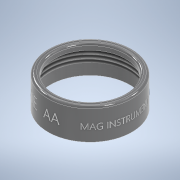
# Autodesk Inventor part: Cap
Saved by Autodesk Inventor 2021 (Build 250183000, 183)
## iProperties
Created: 2020-04-08
Part Number: Cap
Material: Generic
Document SubType Name: Modeling
Designer: Elijah
Density: 1 g/cm^3
Appearance: Silicon Nitride - Polished
Author: Elijah
Autodesk Inventor part; units mm, degrees
ref_plane "XZ Plane" through (0, 0, 0) normal (0, 1, 0) x (-1, 0, 0)
ref_plane "XY Plane" through (0, 0, 0) normal (0, 0, 1) x (1, 0, 0)
sketch "Sketch1" plane through (0, 0, 0) normal (0, 1, 0) x (-1, 0, 0)
  circle A0 centre (0, 0) radius 11.43
  circle A1 centre (0, 0) radius 13.5
  dimension "d0" = 22.86
  dimension "d1" = 27
  constraints: 2 centre point, 2 coincident
  measures "d0" diameter of A0
  measures "d1" diameter of A1
extrude "Extrusion1" add sketch "Sketch1" along normal blind 10
fillet "Fillet1" radius 0.7 2 edges at (13.5, 10, 0) (11.43, 10, 0)
sketch "Sketch2" plane through (0, 0, 0) normal (0, -1, 0) x (1, 0, 0)
  circle A0 centre (0, 0) radius 12.8492
  constraints: 1 centre point, 1 coincident
extrude "Extrusion2" cut sketch "Sketch2" against normal blind 8
ref_plane "Work Plane1" through (13.5, 0, 0) normal (1, 0, 0) x (0, 1, 0)
sketch "Sketch3" plane through (13.5, 0, 0) normal (1, 0, 0) x (0, 1, 0)
  line L0 (7.7302, 43.5284) -> (7.7302, 29.5201) construction
  line L1 (7.7302, 29.5201) -> (-6.2781, 29.5201) construction
  line L2 (-6.2781, 29.5201) -> (-6.2781, 43.5284) construction
  line L3 (-6.2781, 43.5284) -> (7.7302, 43.5284) construction
  line L4 (29.5152, 13.7326) -> (63.5734, 13.7326)
  line L5 (3.4122, 40.2417) -> (5.7555, 40.2417)
  spline S0 degree 2 poles (5.7555, 40.2417) (5.8412, 40.2417) (6.2425, 40.2172) knots 0 0 0 1 1 1
  line L6 (6.2425, 40.2172) -> (6.2425, 40.2264)
  spline S1 degree 2 poles (6.2425, 40.2264) (6.0556, 40.2968) (5.9546, 40.3459) knots 0 0 0 1 1 1
  line L7 (5.9546, 40.3459) -> (3.4122, 41.5221)
  line L8 (3.4122, 41.5221) -> (3.4122, 41.5956)
  line L9 (3.4122, 41.5956) -> (5.9392, 42.7749)
  spline S2 degree 2 poles (5.9392, 42.7749) (6.0618, 42.8331) (6.2517, 42.8821) knots 0 0 0 1 1 1
  line L10 (6.2517, 42.8821) -> (6.2517, 42.8943)
  spline S3 degree 2 poles (6.2517, 42.8943) (6.0311, 42.879) (5.8106, 42.879) knots 0 0 0 1 1 1
  line L11 (5.8106, 42.879) -> (3.4122, 42.879)
  line L12 (3.4122, 42.879) -> (3.4122, 43.1057)
  line L13 (3.4122, 43.1057) -> (6.7142, 43.1057)
  line L14 (6.7142, 43.1057) -> (6.7142, 42.8943)
  line L15 (6.7142, 42.8943) -> (4.0555, 41.663)
  spline S4 degree 2 poles (4.0555, 41.663) (4.0309, 41.6507) (3.9911, 41.6354) knots 0 0 0 1 1 1
  spline S5 degree 2 poles (3.9911, 41.6354) (3.9544, 41.6232) (3.9145, 41.6078) knots 0 0 0 1 1 1
  spline S6 degree 2 poles (3.9145, 41.6078) (3.8533, 41.5833) (3.7798, 41.5588) knots 0 0 0 1 1 1
  line L16 (3.7798, 41.5588) -> (3.7798, 41.5435)
  line L17 (3.7798, 41.5435) -> (3.8533, 41.519)
  spline S7 degree 2 poles (3.8533, 41.519) (3.8625, 41.516) (4.0738, 41.4394) knots 0 0 0 1 1 1
  line L18 (4.0738, 41.4394) -> (6.7142, 40.2264)
  line L19 (6.7142, 40.2264) -> (6.7142, 40.0242)
  line L20 (6.7142, 40.0242) -> (3.4122, 40.0242)
  line L21 (3.4122, 40.0242) -> (3.4122, 40.2417)
  line L22 (3.4122, 37.0194) -> (4.4414, 37.3992)
  line L23 (4.4414, 37.3992) -> (4.4414, 38.8327)
  line L24 (4.4414, 38.8327) -> (3.4122, 39.2125)
  line L25 (3.4122, 39.2125) -> (3.4122, 39.4637)
  line L26 (3.4122, 39.4637) -> (6.7142, 38.217)
  line L27 (6.7142, 38.217) -> (6.7142, 37.9995)
  line L28 (6.7142, 37.9995) -> (3.4122, 36.7651)
  line L29 (3.4122, 36.7651) -> (3.4122, 37.0194)
  spline S8 degree 2 poles (6.1751, 38.0363) (6.2456, 38.0608) (6.3129, 38.0761) knots 0 0 0 1 1 1
  spline S9 degree 2 poles (6.3129, 38.0761) (6.3681, 38.0945) (6.4263, 38.1129) knots 0 0 0 1 1 1
  line L30 (6.4263, 38.1129) -> (6.4263, 38.1221)
  spline S10 degree 2 poles (6.4263, 38.1221) (6.2731, 38.1619) (6.1812, 38.1986) knots 0 0 0 1 1 1
  line L31 (6.1812, 38.1986) -> (4.6497, 38.7531)
  line L32 (4.6497, 38.7531) -> (4.6497, 37.4788)
  line L33 (4.6497, 37.4788) -> (6.1751, 38.0363)
  spline S11 degree 2 poles (3.6419, 33.8184) (3.354, 34.33) (3.354, 34.8721) knots 0 0 0 1 1 1
  spline S12 degree 2 poles (3.354, 34.8721) (3.354, 35.546) (4.2699, 36.3792) (5.0142, 36.3792) knots 0 0 0 1 2 2 2
  spline S13 degree 2 poles (5.0142, 36.3792) (5.7646, 36.3792) (6.7693, 35.4817) (6.7693, 34.7312) knots 0 0 0 1 2 2 2
  spline S14 degree 2 poles (6.7693, 34.7312) (6.7693, 34.2963) (6.5947, 33.8858) knots 0 0 0 1 1 1
  line L34 (6.5947, 33.8858) -> (6.3436, 33.8858)
  spline S15 degree 2 poles (6.3436, 33.8858) (6.561, 34.333) (6.561, 34.7619) knots 0 0 0 1 1 1
  spline S16 degree 2 poles (6.561, 34.7619) (6.561, 35.3867) (5.7095, 36.1433) (5.0479, 36.1433) knots 0 0 0 1 2 2 2
  spline S17 degree 2 poles (5.0479, 36.1433) (4.3526, 36.1433) (3.5623, 35.4327) (3.5623, 34.8293) knots 0 0 0 1 2 2 2
  spline S18 degree 2 poles (3.5623, 34.8293) (3.5623, 34.382) (3.7553, 34.0451) knots 0 0 0 1 1 1
  line L35 (3.7553, 34.0451) -> (4.8457, 34.0451)
  line L36 (4.8457, 34.0451) -> (4.8457, 34.8231)
  line L37 (4.8457, 34.8231) -> (5.054, 34.8231)
  line L38 (5.054, 34.8231) -> (5.054, 33.8184)
  line L39 (5.054, 33.8184) -> (3.6419, 33.8184)
  line L40 (3.4122, 33.0557) -> (6.7142, 33.0557)
  line L41 (6.7142, 33.0557) -> (6.7142, 32.8291)
  line L42 (6.7142, 32.8291) -> (3.6205, 32.8291)
  line L43 (3.6205, 32.8291) -> (3.6205, 31.5027)
  line L44 (3.6205, 31.5027) -> (3.4122, 31.5027)
  line L45 (3.4122, 31.5027) -> (3.4122, 33.0557)
  line L46 (3.4122, 30.8963) -> (6.7142, 30.8963)
  line L47 (6.7142, 30.8963) -> (6.7142, 30.6696)
  line L48 (6.7142, 30.6696) -> (3.4122, 30.6696)
  line L49 (3.4122, 30.6696) -> (3.4122, 30.8963)
  line L50 (6.5059, 28.9236) -> (3.4122, 28.9236)
  line L51 (3.4122, 28.9236) -> (3.4122, 29.1503)
  line L52 (3.4122, 29.1503) -> (6.5059, 29.1503)
  line L53 (6.5059, 29.1503) -> (6.5059, 30.1029)
  line L54 (6.5059, 30.1029) -> (6.7142, 30.1029)
  line L55 (6.7142, 30.1029) -> (6.7142, 27.971)
  line L56 (6.7142, 27.971) -> (6.5059, 27.971)
  line L57 (6.5059, 27.971) -> (6.5059, 28.9236)
  line L58 (3.4122, 27.4105) -> (6.7142, 27.4105)
  line L59 (6.7142, 27.4105) -> (6.7142, 25.8667)
  line L60 (6.7142, 25.8667) -> (6.5059, 25.8667)
  line L61 (6.5059, 25.8667) -> (6.5059, 27.1838)
  line L62 (6.5059, 27.1838) -> (5.1796, 27.1838)
  line L63 (5.1796, 27.1838) -> (5.1796, 25.9616)
  line L64 (5.1796, 25.9616) -> (4.9713, 25.9616)
  line L65 (4.9713, 25.9616) -> (4.9713, 27.1838)
  line L66 (4.9713, 27.1838) -> (3.6205, 27.1838)
  line L67 (3.6205, 27.1838) -> (3.6205, 25.7901)
  line L68 (3.6205, 25.7901) -> (3.4122, 25.7901)
  line L69 (3.4122, 25.7901) -> (3.4122, 27.4105)
  line L70 (3.4122, 20.707) -> (4.2831, 21.0284)
  line L71 (4.2831, 21.0284) -> (4.2831, 22.2414)
  line L72 (4.2831, 22.2414) -> (3.4122, 22.5628)
  line L73 (3.4122, 22.5628) -> (3.4122, 22.7753)
  line L74 (3.4122, 22.7753) -> (6.2062, 21.7204)
  line L75 (6.2062, 21.7204) -> (6.2062, 21.5364)
  line L76 (6.2062, 21.5364) -> (3.4122, 20.4919)
  line L77 (3.4122, 20.4919) -> (3.4122, 20.707)
  spline S19 degree 2 poles (5.75, 21.5675) (5.8097, 21.5883) (5.8667, 21.6012) knots 0 0 0 1 1 1
  spline S20 degree 2 poles (5.8667, 21.6012) (5.9133, 21.6168) (5.9626, 21.6323) knots 0 0 0 1 1 1
  line L78 (5.9626, 21.6323) -> (5.9626, 21.6401)
  spline S21 degree 2 poles (5.9626, 21.6401) (5.833, 21.6738) (5.7552, 21.7049) knots 0 0 0 1 1 1
  line L79 (5.7552, 21.7049) -> (4.4593, 22.174)
  line L80 (4.4593, 22.174) -> (4.4593, 21.0958)
  line L81 (4.4593, 21.0958) -> (5.75, 21.5675)
  line L82 (3.4122, 18.1955) -> (4.2831, 18.5169)
  line L83 (4.2831, 18.5169) -> (4.2831, 19.7299)
  line L84 (4.2831, 19.7299) -> (3.4122, 20.0513)
  line L85 (3.4122, 20.0513) -> (3.4122, 20.2638)
  line L86 (3.4122, 20.2638) -> (6.2062, 19.209)
  line L87 (6.2062, 19.209) -> (6.2062, 19.0249)
  line L88 (6.2062, 19.0249) -> (3.4122, 17.9804)
  line L89 (3.4122, 17.9804) -> (3.4122, 18.1955)
  spline S22 degree 2 poles (5.75, 19.056) (5.8097, 19.0768) (5.8667, 19.0897) knots 0 0 0 1 1 1
  spline S23 degree 2 poles (5.8667, 19.0897) (5.9133, 19.1053) (5.9626, 19.1208) knots 0 0 0 1 1 1
  line L90 (5.9626, 19.1208) -> (5.9626, 19.1286)
  spline S24 degree 2 poles (5.9626, 19.1286) (5.833, 19.1623) (5.7552, 19.1934) knots 0 0 0 1 1 1
  line L91 (5.7552, 19.1934) -> (4.4593, 19.6625)
  line L92 (4.4593, 19.6625) -> (4.4593, 18.5843)
  line L93 (4.4593, 18.5843) -> (5.75, 19.056)
  line L94 (3.4122, 11.125) -> (4.674, 11.125)
  spline S25 degree 2 poles (4.674, 11.125) (4.7201, 11.125) (4.9362, 11.1118) knots 0 0 0 1 1 1
  line L95 (4.9362, 11.1118) -> (4.9362, 11.1168)
  spline S26 degree 2 poles (4.9362, 11.1168) (4.8356, 11.1547) (4.7812, 11.1811) knots 0 0 0 1 1 1
  line L96 (4.7812, 11.1811) -> (3.4122, 11.8144)
  line L97 (3.4122, 11.8144) -> (3.4122, 11.854)
  line L98 (3.4122, 11.854) -> (4.7729, 12.489)
  spline S27 degree 2 poles (4.7729, 12.489) (4.8389, 12.5204) (4.9412, 12.5468) knots 0 0 0 1 1 1
  line L99 (4.9412, 12.5468) -> (4.9412, 12.5534)
  spline S28 degree 2 poles (4.9412, 12.5534) (4.8224, 12.5451) (4.7036, 12.5451) knots 0 0 0 1 1 1
  line L100 (4.7036, 12.5451) -> (3.4122, 12.5451)
  line L101 (3.4122, 12.5451) -> (3.4122, 12.6672)
  line L102 (3.4122, 12.6672) -> (5.1902, 12.6672)
  line L103 (5.1902, 12.6672) -> (5.1902, 12.5534)
  line L104 (5.1902, 12.5534) -> (3.7586, 11.8903)
  spline S29 degree 2 poles (3.7586, 11.8903) (3.7454, 11.8837) (3.7239, 11.8755) knots 0 0 0 1 1 1
  spline S30 degree 2 poles (3.7239, 11.8755) (3.7041, 11.8689) (3.6827, 11.8606) knots 0 0 0 1 1 1
  spline S31 degree 2 poles (3.6827, 11.8606) (3.6497, 11.8474) (3.6101, 11.8342) knots 0 0 0 1 1 1
  line L105 (3.6101, 11.8342) -> (3.6101, 11.826)
  line L106 (3.6101, 11.826) -> (3.6497, 11.8128)
  spline S32 degree 2 poles (3.6497, 11.8128) (3.6547, 11.8111) (3.7685, 11.7699) knots 0 0 0 1 1 1
  line L107 (3.7685, 11.7699) -> (5.1902, 11.1168)
  line L108 (5.1902, 11.1168) -> (5.1902, 11.0079)
  line L109 (5.1902, 11.0079) -> (3.4122, 11.0079)
  line L110 (3.4122, 11.0079) -> (3.4122, 11.125)
  line L111 (3.4122, 9.3899) -> (3.9664, 9.5944)
  line L112 (3.9664, 9.5944) -> (3.9664, 10.3663)
  line L113 (3.9664, 10.3663) -> (3.4122, 10.5708)
  line L114 (3.4122, 10.5708) -> (3.4122, 10.7061)
  line L115 (3.4122, 10.7061) -> (5.1902, 10.0348)
  line L116 (5.1902, 10.0348) -> (5.1902, 9.9177)
  line L117 (5.1902, 9.9177) -> (3.4122, 9.253)
  line L118 (3.4122, 9.253) -> (3.4122, 9.3899)
  spline S33 degree 2 poles (4.8999, 9.9375) (4.9379, 9.9507) (4.9741, 9.9589) knots 0 0 0 1 1 1
  spline S34 degree 2 poles (4.9741, 9.9589) (5.0038, 9.9688) (5.0352, 9.9787) knots 0 0 0 1 1 1
  line L119 (5.0352, 9.9787) -> (5.0352, 9.9837)
  spline S35 degree 2 poles (5.0352, 9.9837) (4.9527, 10.0051) (4.9032, 10.0249) knots 0 0 0 1 1 1
  line L120 (4.9032, 10.0249) -> (4.0785, 10.3234)
  line L121 (4.0785, 10.3234) -> (4.0785, 9.6373)
  line L122 (4.0785, 9.6373) -> (4.8999, 9.9375)
  spline S36 degree 2 poles (3.5359, 7.6663) (3.3809, 7.9418) (3.3809, 8.2337) knots 0 0 0 1 1 1
  spline S37 degree 2 poles (3.3809, 8.2337) (3.3809, 8.5966) (3.874, 9.0452) (4.2748, 9.0452) knots 0 0 0 1 2 2 2
  spline S38 degree 2 poles (4.2748, 9.0452) (4.6789, 9.0452) (5.2199, 8.5619) (5.2199, 8.1578) knots 0 0 0 1 2 2 2
  spline S39 degree 2 poles (5.2199, 8.1578) (5.2199, 7.9236) (5.1259, 7.7026) knots 0 0 0 1 1 1
  line L123 (5.1259, 7.7026) -> (4.9906, 7.7026)
  spline S40 degree 2 poles (4.9906, 7.7026) (5.1077, 7.9434) (5.1077, 8.1743) knots 0 0 0 1 1 1
  spline S41 degree 2 poles (5.1077, 8.1743) (5.1077, 8.5108) (4.6492, 8.9182) (4.293, 8.9182) knots 0 0 0 1 2 2 2
  spline S42 degree 2 poles (4.293, 8.9182) (3.9186, 8.9182) (3.493, 8.5355) (3.493, 8.2106) knots 0 0 0 1 2 2 2
  spline S43 degree 2 poles (3.493, 8.2106) (3.493, 7.9698) (3.5969, 7.7884) knots 0 0 0 1 1 1
  line L124 (3.5969, 7.7884) -> (4.1841, 7.7884)
  line L125 (4.1841, 7.7884) -> (4.1841, 8.2073)
  line L126 (4.1841, 8.2073) -> (4.2963, 8.2073)
  line L127 (4.2963, 8.2073) -> (4.2963, 7.6663)
  line L128 (4.2963, 7.6663) -> (3.5359, 7.6663)
  line L129 (3.4122, 6.5596) -> (5.1902, 6.5596)
  line L130 (5.1902, 6.5596) -> (5.1902, 6.4376)
  line L131 (5.1902, 6.4376) -> (3.4122, 6.4376)
  line L132 (3.4122, 6.4376) -> (3.4122, 6.5596)
  line L133 (3.4122, 4.7222) -> (4.8488, 5.7828)
  spline S44 degree 2 poles (4.8488, 5.7828) (4.8933, 5.8158) (4.9362, 5.8405) knots 0 0 0 1 1 1
  line L134 (4.9362, 5.8405) -> (4.9609, 5.8553)
  line L135 (4.9609, 5.8553) -> (4.9609, 5.8603)
  spline S45 degree 2 poles (4.9609, 5.8603) (4.928, 5.8586) (4.8834, 5.8586) knots 0 0 0 1 1 1
  line L136 (4.8834, 5.8586) -> (3.4122, 5.8586)
  line L137 (3.4122, 5.8586) -> (3.4122, 5.9807)
  line L138 (3.4122, 5.9807) -> (5.1902, 5.9807)
  line L139 (5.1902, 5.9807) -> (5.1902, 5.8867)
  line L140 (5.1902, 5.8867) -> (3.7652, 4.8344)
  spline S46 degree 2 poles (3.7652, 4.8344) (3.719, 4.7998) (3.6514, 4.7585) knots 0 0 0 1 1 1
  line L141 (3.6514, 4.7585) -> (3.6514, 4.7519)
  spline S47 degree 2 poles (3.6514, 4.7519) (3.7388, 4.7585) (3.7998, 4.7585) knots 0 0 0 1 1 1
  line L142 (3.7998, 4.7585) -> (5.1902, 4.7585)
  line L143 (5.1902, 4.7585) -> (5.1902, 4.6365)
  line L144 (5.1902, 4.6365) -> (3.4122, 4.6365)
  line L145 (3.4122, 4.6365) -> (3.4122, 4.7222)
  line L146 (3.4749, 4.234) -> (3.6151, 4.234)
  spline S48 degree 2 poles (3.6151, 4.234) (3.493, 4.0427) (3.493, 3.8481) knots 0 0 0 1 1 1
  spline S49 degree 2 poles (3.493, 3.8481) (3.493, 3.6403) (3.6662, 3.4242) (3.8212, 3.4242) knots 0 0 0 1 2 2 2
  spline S50 degree 2 poles (3.8212, 3.4242) (3.9581, 3.4242) (4.1198, 3.5693) (4.26, 3.8101) knots 0 0 0 1 2 2 2
  spline S51 degree 2 poles (4.26, 3.8101) (4.4183, 4.0806) (4.6294, 4.2241) (4.768, 4.2241) knots 0 0 0 1 2 2 2
  spline S52 degree 2 poles (4.768, 4.2241) (4.9576, 4.2241) (5.2199, 3.9322) (5.2199, 3.6864) knots 0 0 0 1 2 2 2
  spline S53 degree 2 poles (5.2199, 3.6864) (5.2199, 3.5281) (5.1671, 3.3698) knots 0 0 0 1 1 1
  line L147 (5.1671, 3.3698) -> (5.0368, 3.3698)
  spline S54 degree 2 poles (5.0368, 3.3698) (5.1077, 3.5265) (5.1077, 3.7029) knots 0 0 0 1 1 1
  spline S55 degree 2 poles (5.1077, 3.7029) (5.1077, 3.8844) (4.9247, 4.0971) (4.7828, 4.0971) knots 0 0 0 1 2 2 2
  spline S56 degree 2 poles (4.7828, 4.0971) (4.6476, 4.0971) (4.4859, 3.952) (4.3474, 3.7112) knots 0 0 0 1 2 2 2
  spline S57 degree 2 poles (4.3474, 3.7112) (4.2055, 3.4621) (3.9862, 3.2972) (3.8427, 3.2972) knots 0 0 0 1 2 2 2
  spline S58 degree 2 poles (3.8427, 3.2972) (3.6382, 3.2972) (3.3809, 3.5809) (3.3809, 3.8398) knots 0 0 0 1 2 2 2
  spline S59 degree 2 poles (3.3809, 3.8398) (3.3809, 3.9322) (3.4369, 4.1714) (3.4749, 4.234) knots 0 0 0 1 2 2 2
  line L148 (5.078, 2.4346) -> (3.4122, 2.4346)
  line L149 (3.4122, 2.4346) -> (3.4122, 2.5566)
  line L150 (3.4122, 2.5566) -> (5.078, 2.5566)
  line L151 (5.078, 2.5566) -> (5.078, 3.0696)
  line L152 (5.078, 3.0696) -> (5.1902, 3.0696)
  line L153 (5.1902, 3.0696) -> (5.1902, 1.9216)
  line L154 (5.1902, 1.9216) -> (5.078, 1.9216)
  line L155 (5.078, 1.9216) -> (5.078, 2.4346)
  line L156 (3.4122, 0.7094) -> (3.9334, 0.9469)
  spline S60 degree 2 poles (3.9334, 0.9469) (4.0934, 1.0194) (4.2039, 1.1662) (4.2039, 1.2767) knots 0 0 0 1 2 2 2
  line L157 (4.2039, 1.2767) -> (4.2039, 1.4978)
  line L158 (4.2039, 1.4978) -> (3.4122, 1.4978)
  line L159 (3.4122, 1.4978) -> (3.4122, 1.6198)
  line L160 (3.4122, 1.6198) -> (5.1902, 1.6198)
  line L161 (5.1902, 1.6198) -> (5.1902, 1.125)
  spline S61 degree 2 poles (5.1902, 1.125) (5.1902, 0.8891) (4.9362, 0.6203) (4.7267, 0.6203) knots 0 0 0 1 2 2 2
  spline S62 degree 2 poles (4.7267, 0.6203) (4.5354, 0.6203) (4.2765, 0.8413) (4.2402, 1.0409) knots 0 0 0 1 2 2 2
  line L162 (4.2402, 1.0409) -> (4.2352, 1.0409)
  spline S63 degree 2 poles (4.2352, 1.0409) (4.1923, 0.9353) (3.9779, 0.8347) knots 0 0 0 1 1 1
  line L163 (3.9779, 0.8347) -> (3.4122, 0.5692)
  line L164 (3.4122, 0.5692) -> (3.4122, 0.7094)
  line L165 (5.078, 1.4978) -> (4.316, 1.4978)
  line L166 (4.316, 1.4978) -> (4.316, 1.191)
  spline S64 degree 2 poles (4.316, 1.191) (4.316, 0.9865) (4.5288, 0.7473) (4.7152, 0.7473) knots 0 0 0 1 2 2 2
  spline S65 degree 2 poles (4.7152, 0.7473) (4.8851, 0.7473) (5.078, 0.9634) (5.078, 1.1646) knots 0 0 0 1 2 2 2
  line L167 (5.078, 1.1646) -> (5.078, 1.4978)
  spline S66 degree 2 poles (4.1231, -1.0027) (3.3809, -1.0027) (3.3809, -0.371) knots 0 0 0 1 1 1
  spline S67 degree 2 poles (3.3809, -0.371) (3.3809, 0.2311) (4.095, 0.2311) knots 0 0 0 1 1 1
  line L168 (4.095, 0.2311) -> (5.1902, 0.2311)
  line L169 (5.1902, 0.2311) -> (5.1902, 0.109)
  line L170 (5.1902, 0.109) -> (4.1115, 0.109)
  spline S68 degree 2 poles (4.1115, 0.109) (3.493, 0.109) (3.493, -0.394) knots 0 0 0 1 1 1
  spline S69 degree 2 poles (3.493, -0.394) (3.493, -0.8806) (4.095, -0.8806) knots 0 0 0 1 1 1
  line L171 (4.095, -0.8806) -> (5.1902, -0.8806)
  line L172 (5.1902, -0.8806) -> (5.1902, -1.0027)
  line L173 (5.1902, -1.0027) -> (4.1231, -1.0027)
  line L174 (3.4122, -2.9786) -> (4.674, -2.9786)
  spline S70 degree 2 poles (4.674, -2.9786) (4.7201, -2.9786) (4.9362, -2.9918) knots 0 0 0 1 1 1
  line L175 (4.9362, -2.9918) -> (4.9362, -2.9868)
  spline S71 degree 2 poles (4.9362, -2.9868) (4.8356, -2.9489) (4.7812, -2.9225) knots 0 0 0 1 1 1
  line L176 (4.7812, -2.9225) -> (3.4122, -2.2891)
  line L177 (3.4122, -2.2891) -> (3.4122, -2.2496)
  line L178 (3.4122, -2.2496) -> (4.7729, -1.6146)
  spline S72 degree 2 poles (4.7729, -1.6146) (4.8389, -1.5832) (4.9412, -1.5568) knots 0 0 0 1 1 1
  line L179 (4.9412, -1.5568) -> (4.9412, -1.5502)
  spline S73 degree 2 poles (4.9412, -1.5502) (4.8224, -1.5585) (4.7036, -1.5585) knots 0 0 0 1 1 1
  line L180 (4.7036, -1.5585) -> (3.4122, -1.5585)
  line L181 (3.4122, -1.5585) -> (3.4122, -1.4364)
  line L182 (3.4122, -1.4364) -> (5.1902, -1.4364)
  line L183 (5.1902, -1.4364) -> (5.1902, -1.5502)
  line L184 (5.1902, -1.5502) -> (3.7586, -2.2133)
  spline S74 degree 2 poles (3.7586, -2.2133) (3.7454, -2.2199) (3.7239, -2.2281) knots 0 0 0 1 1 1
  spline S75 degree 2 poles (3.7239, -2.2281) (3.7041, -2.2347) (3.6827, -2.243) knots 0 0 0 1 1 1
  spline S76 degree 2 poles (3.6827, -2.243) (3.6497, -2.2562) (3.6101, -2.2694) knots 0 0 0 1 1 1
  line L185 (3.6101, -2.2694) -> (3.6101, -2.2776)
  line L186 (3.6101, -2.2776) -> (3.6497, -2.2908)
  spline S77 degree 2 poles (3.6497, -2.2908) (3.6547, -2.2924) (3.7685, -2.3337) knots 0 0 0 1 1 1
  line L187 (3.7685, -2.3337) -> (5.1902, -2.9868)
  line L188 (5.1902, -2.9868) -> (5.1902, -3.0957)
  line L189 (5.1902, -3.0957) -> (3.4122, -3.0957)
  line L190 (3.4122, -3.0957) -> (3.4122, -2.9786)
  line L191 (3.4122, -3.5526) -> (5.1902, -3.5526)
  line L192 (5.1902, -3.5526) -> (5.1902, -4.3838)
  line L193 (5.1902, -4.3838) -> (5.078, -4.3838)
  line L194 (5.078, -4.3838) -> (5.078, -3.6746)
  line L195 (5.078, -3.6746) -> (4.3639, -3.6746)
  line L196 (4.3639, -3.6746) -> (4.3639, -4.3327)
  line L197 (4.3639, -4.3327) -> (4.2517, -4.3327)
  line L198 (4.2517, -4.3327) -> (4.2517, -3.6746)
  line L199 (4.2517, -3.6746) -> (3.5244, -3.6746)
  line L200 (3.5244, -3.6746) -> (3.5244, -4.4251)
  line L201 (3.5244, -4.4251) -> (3.4122, -4.4251)
  line L202 (3.4122, -4.4251) -> (3.4122, -3.5526)
  line L203 (3.4122, -6.081) -> (4.8488, -5.0205)
  spline S78 degree 2 poles (4.8488, -5.0205) (4.8933, -4.9875) (4.9362, -4.9627) knots 0 0 0 1 1 1
  line L204 (4.9362, -4.9627) -> (4.9609, -4.9479)
  line L205 (4.9609, -4.9479) -> (4.9609, -4.943)
  spline S79 degree 2 poles (4.9609, -4.943) (4.928, -4.9446) (4.8834, -4.9446) knots 0 0 0 1 1 1
  line L206 (4.8834, -4.9446) -> (3.4122, -4.9446)
  line L207 (3.4122, -4.9446) -> (3.4122, -4.8226)
  line L208 (3.4122, -4.8226) -> (5.1902, -4.8226)
  line L209 (5.1902, -4.8226) -> (5.1902, -4.9166)
  line L210 (5.1902, -4.9166) -> (3.7652, -5.9689)
  spline S80 degree 2 poles (3.7652, -5.9689) (3.719, -6.0035) (3.6514, -6.0447) knots 0 0 0 1 1 1
  line L211 (3.6514, -6.0447) -> (3.6514, -6.0513)
  spline S81 degree 2 poles (3.6514, -6.0513) (3.7388, -6.0447) (3.7998, -6.0447) knots 0 0 0 1 1 1
  line L212 (3.7998, -6.0447) -> (5.1902, -6.0447)
  line L213 (5.1902, -6.0447) -> (5.1902, -6.1668)
  line L214 (5.1902, -6.1668) -> (3.4122, -6.1668)
  line L215 (3.4122, -6.1668) -> (3.4122, -6.081)
  line L216 (5.078, -7.1069) -> (3.4122, -7.1069)
  line L217 (3.4122, -7.1069) -> (3.4122, -6.9849)
  line L218 (3.4122, -6.9849) -> (5.078, -6.9849)
  line L219 (5.078, -6.9849) -> (5.078, -6.4719)
  line L220 (5.078, -6.4719) -> (5.1902, -6.4719)
  line L221 (5.1902, -6.4719) -> (5.1902, -7.6199)
  line L222 (5.1902, -7.6199) -> (5.078, -7.6199)
  line L223 (5.078, -7.6199) -> (5.078, -7.1069)
  line L224 (4.1, -8.5699) -> (4.2121, -8.5699)
  line L225 (4.2121, -8.5699) -> (4.2121, -9.2478)
  line L226 (4.2121, -9.2478) -> (4.1, -9.2478)
  line L227 (4.1, -9.2478) -> (4.1, -8.5699)
  spline S82 degree 2 poles (3.4699, -11.5074) (3.3809, -11.2913) (3.3809, -11.0571) knots 0 0 0 1 1 1
  spline S83 degree 2 poles (3.3809, -11.0571) (3.3809, -10.6926) (3.8707, -10.2324) (4.2649, -10.2324) knots 0 0 0 1 2 2 2
  spline S84 degree 2 poles (4.2649, -10.2324) (4.697, -10.2324) (5.2199, -10.7305) (5.2199, -11.1148) knots 0 0 0 1 2 2 2
  spline S85 degree 2 poles (5.2199, -11.1148) (5.2199, -11.3193) (5.1539, -11.5074) knots 0 0 0 1 1 1
  line L228 (5.1539, -11.5074) -> (5.0236, -11.5074)
  spline S86 degree 2 poles (5.0236, -11.5074) (5.1077, -11.321) (5.1077, -11.1132) knots 0 0 0 1 1 1
  spline S87 degree 2 poles (5.1077, -11.1132) (5.1077, -10.7784) (4.6542, -10.3594) (4.2765, -10.3594) knots 0 0 0 1 2 2 2
  spline S88 degree 2 poles (4.2765, -10.3594) (3.9136, -10.3594) (3.493, -10.7602) (3.493, -11.067) knots 0 0 0 1 2 2 2
  spline S89 degree 2 poles (3.493, -11.067) (3.493, -11.3127) (3.5887, -11.5074) knots 0 0 0 1 1 1
  line L229 (3.5887, -11.5074) -> (3.4699, -11.5074)
  line L230 (3.4122, -13.0627) -> (3.9664, -12.8582)
  line L231 (3.9664, -12.8582) -> (3.9664, -12.0863)
  line L232 (3.9664, -12.0863) -> (3.4122, -11.8818)
  line L233 (3.4122, -11.8818) -> (3.4122, -11.7465)
  line L234 (3.4122, -11.7465) -> (5.1902, -12.4178)
  line L235 (5.1902, -12.4178) -> (5.1902, -12.5349)
  line L236 (5.1902, -12.5349) -> (3.4122, -13.1996)
  line L237 (3.4122, -13.1996) -> (3.4122, -13.0627)
  spline S90 degree 2 poles (4.8999, -12.5151) (4.9379, -12.5019) (4.9741, -12.4937) knots 0 0 0 1 1 1
  spline S91 degree 2 poles (4.9741, -12.4937) (5.0038, -12.4838) (5.0352, -12.4739) knots 0 0 0 1 1 1
  line L238 (5.0352, -12.4739) -> (5.0352, -12.4689)
  spline S92 degree 2 poles (5.0352, -12.4689) (4.9527, -12.4475) (4.9032, -12.4277) knots 0 0 0 1 1 1
  line L239 (4.9032, -12.4277) -> (4.0785, -12.1292)
  line L240 (4.0785, -12.1292) -> (4.0785, -12.8153)
  line L241 (4.0785, -12.8153) -> (4.8999, -12.5151)
  line L242 (3.4122, -13.4998) -> (5.1902, -13.4998)
  line L243 (5.1902, -13.4998) -> (5.1902, -13.6218)
  line L244 (5.1902, -13.6218) -> (3.5244, -13.6218)
  line L245 (3.5244, -13.6218) -> (3.5244, -14.336)
  line L246 (3.5244, -14.336) -> (3.4122, -14.336)
  line L247 (3.4122, -14.336) -> (3.4122, -13.4998)
  line L248 (3.4122, -14.6626) -> (5.1902, -14.6626)
  line L249 (5.1902, -14.6626) -> (5.1902, -14.7846)
  line L250 (5.1902, -14.7846) -> (3.4122, -14.7846)
  line L251 (3.4122, -14.7846) -> (3.4122, -14.6626)
  line L252 (5.078, -15.3636) -> (4.3523, -15.3636)
  line L253 (4.3523, -15.3636) -> (4.3523, -16.0216)
  line L254 (4.3523, -16.0216) -> (4.2402, -16.0216)
  line L255 (4.2402, -16.0216) -> (4.2402, -15.3636)
  line L256 (4.2402, -15.3636) -> (3.4122, -15.3636)
  line L257 (3.4122, -15.3636) -> (3.4122, -15.2415)
  line L258 (3.4122, -15.2415) -> (5.1902, -15.2415)
  line L259 (5.1902, -15.2415) -> (5.1902, -16.0728)
  line L260 (5.1902, -16.0728) -> (5.078, -16.0728)
  line L261 (5.078, -16.0728) -> (5.078, -15.3636)
  spline S93 degree 2 poles (3.3809, -17.1547) (3.3809, -16.7787) (3.8823, -16.3301) (4.2831, -16.3301) knots 0 0 0 1 2 2 2
  spline S94 degree 2 poles (4.2831, -16.3301) (4.7069, -16.3301) (5.2199, -16.7902) (5.2199, -17.1894) knots 0 0 0 1 2 2 2
  spline S95 degree 2 poles (5.2199, -17.1894) (5.2199, -17.5489) (4.7284, -17.9943) (4.3276, -17.9943) knots 0 0 0 1 2 2 2
  spline S96 degree 2 poles (4.3276, -17.9943) (3.8872, -17.9943) (3.3809, -17.5374) (3.3809, -17.1547) knots 0 0 0 1 2 2 2
  spline S97 degree 2 poles (5.1077, -17.1679) (5.1077, -16.8579) (4.6591, -16.4571) (4.2963, -16.4571) knots 0 0 0 1 2 2 2
  spline S98 degree 2 poles (4.2963, -16.4571) (3.9285, -16.4571) (3.493, -16.8364) (3.493, -17.1531) knots 0 0 0 1 2 2 2
  spline S99 degree 2 poles (3.493, -17.1531) (3.493, -17.483) (3.9235, -17.8673) (4.3078, -17.8673) knots 0 0 0 1 2 2 2
  spline S100 degree 2 poles (4.3078, -17.8673) (4.6855, -17.8673) (5.1077, -17.4912) (5.1077, -17.1679) knots 0 0 0 1 2 2 2
  line L262 (3.4122, -19.2659) -> (3.9334, -19.0284)
  spline S101 degree 2 poles (3.9334, -19.0284) (4.0934, -18.9558) (4.2039, -18.809) (4.2039, -18.6985) knots 0 0 0 1 2 2 2
  line L263 (4.2039, -18.6985) -> (4.2039, -18.4775)
  line L264 (4.2039, -18.4775) -> (3.4122, -18.4775)
  line L265 (3.4122, -18.4775) -> (3.4122, -18.3555)
  line L266 (3.4122, -18.3555) -> (5.1902, -18.3555)
  line L267 (5.1902, -18.3555) -> (5.1902, -18.8503)
  spline S102 degree 2 poles (5.1902, -18.8503) (5.1902, -19.0861) (4.9362, -19.355) (4.7267, -19.355) knots 0 0 0 1 2 2 2
  spline S103 degree 2 poles (4.7267, -19.355) (4.5354, -19.355) (4.2765, -19.134) (4.2402, -18.9344) knots 0 0 0 1 2 2 2
  line L268 (4.2402, -18.9344) -> (4.2352, -18.9344)
  spline S104 degree 2 poles (4.2352, -18.9344) (4.1923, -19.04) (3.9779, -19.1406) knots 0 0 0 1 1 1
  line L269 (3.9779, -19.1406) -> (3.4122, -19.4061)
  line L270 (3.4122, -19.4061) -> (3.4122, -19.2659)
  line L271 (5.078, -18.4775) -> (4.316, -18.4775)
  line L272 (4.316, -18.4775) -> (4.316, -18.7843)
  spline S105 degree 2 poles (4.316, -18.7843) (4.316, -18.9888) (4.5288, -19.228) (4.7152, -19.228) knots 0 0 0 1 2 2 2
  spline S106 degree 2 poles (4.7152, -19.228) (4.8851, -19.228) (5.078, -19.0119) (5.078, -18.8107) knots 0 0 0 1 2 2 2
  line L273 (5.078, -18.8107) -> (5.078, -18.4775)
  line L274 (3.4122, -21.0241) -> (4.8488, -19.9636)
  spline S107 degree 2 poles (4.8488, -19.9636) (4.8933, -19.9306) (4.9362, -19.9059) knots 0 0 0 1 1 1
  line L275 (4.9362, -19.9059) -> (4.9609, -19.891)
  line L276 (4.9609, -19.891) -> (4.9609, -19.8861)
  spline S108 degree 2 poles (4.9609, -19.8861) (4.928, -19.8877) (4.8834, -19.8877) knots 0 0 0 1 1 1
  line L277 (4.8834, -19.8877) -> (3.4122, -19.8877)
  line L278 (3.4122, -19.8877) -> (3.4122, -19.7657)
  line L279 (3.4122, -19.7657) -> (5.1902, -19.7657)
  line L280 (5.1902, -19.7657) -> (5.1902, -19.8597)
  line L281 (5.1902, -19.8597) -> (3.7652, -20.912)
  spline S109 degree 2 poles (3.7652, -20.912) (3.719, -20.9466) (3.6514, -20.9878) knots 0 0 0 1 1 1
  line L282 (3.6514, -20.9878) -> (3.6514, -20.9944)
  spline S110 degree 2 poles (3.6514, -20.9944) (3.7388, -20.9878) (3.7998, -20.9878) knots 0 0 0 1 1 1
  line L283 (3.7998, -20.9878) -> (5.1902, -20.9878)
  line L284 (5.1902, -20.9878) -> (5.1902, -21.1099)
  line L285 (5.1902, -21.1099) -> (3.4122, -21.1099)
  line L286 (3.4122, -21.1099) -> (3.4122, -21.0241)
  line L287 (3.4122, -21.5668) -> (5.1902, -21.5668)
  line L288 (5.1902, -21.5668) -> (5.1902, -21.6888)
  line L289 (5.1902, -21.6888) -> (3.4122, -21.6888)
  line L290 (3.4122, -21.6888) -> (3.4122, -21.5668)
  line L291 (3.4122, -23.3068) -> (3.9664, -23.1023)
  line L292 (3.9664, -23.1023) -> (3.9664, -22.3304)
  line L293 (3.9664, -22.3304) -> (3.4122, -22.1259)
  line L294 (3.4122, -22.1259) -> (3.4122, -21.9906)
  line L295 (3.4122, -21.9906) -> (5.1902, -22.6619)
  line L296 (5.1902, -22.6619) -> (5.1902, -22.779)
  line L297 (5.1902, -22.779) -> (3.4122, -23.4437)
  line L298 (3.4122, -23.4437) -> (3.4122, -23.3068)
  spline S111 degree 2 poles (4.8999, -22.7592) (4.9379, -22.746) (4.9741, -22.7378) knots 0 0 0 1 1 1
  spline S112 degree 2 poles (4.9741, -22.7378) (5.0038, -22.7279) (5.0352, -22.718) knots 0 0 0 1 1 1
  line L299 (5.0352, -22.718) -> (5.0352, -22.7131)
  spline S113 degree 2 poles (5.0352, -22.7131) (4.9527, -22.6916) (4.9032, -22.6718) knots 0 0 0 1 1 1
  line L300 (4.9032, -22.6718) -> (4.0785, -22.3733)
  line L301 (4.0785, -22.3733) -> (4.0785, -23.0594)
  line L302 (4.0785, -23.0594) -> (4.8999, -22.7592)
  spline S114 degree 2 poles (4.1231, -25.6522) (3.3809, -25.6522) (3.3809, -25.0205) knots 0 0 0 1 1 1
  spline S115 degree 2 poles (3.3809, -25.0205) (3.3809, -24.4185) (4.095, -24.4185) knots 0 0 0 1 1 1
  line L303 (4.095, -24.4185) -> (5.1902, -24.4185)
  line L304 (5.1902, -24.4185) -> (5.1902, -24.5405)
  line L305 (5.1902, -24.5405) -> (4.1115, -24.5405)
  spline S116 degree 2 poles (4.1115, -24.5405) (3.493, -24.5405) (3.493, -25.0436) knots 0 0 0 1 1 1
  spline S117 degree 2 poles (3.493, -25.0436) (3.493, -25.5301) (4.095, -25.5301) knots 0 0 0 1 1 1
  line L306 (4.095, -25.5301) -> (5.1902, -25.5301)
  line L307 (5.1902, -25.5301) -> (5.1902, -25.6522)
  line L308 (5.1902, -25.6522) -> (4.1231, -25.6522)
  line L309 (3.4749, -26.0316) -> (3.6151, -26.0316)
  spline S118 degree 2 poles (3.6151, -26.0316) (3.493, -26.2229) (3.493, -26.4175) knots 0 0 0 1 1 1
  spline S119 degree 2 poles (3.493, -26.4175) (3.493, -26.6253) (3.6662, -26.8414) (3.8212, -26.8414) knots 0 0 0 1 2 2 2
  spline S120 degree 2 poles (3.8212, -26.8414) (3.9581, -26.8414) (4.1198, -26.6962) (4.26, -26.4554) knots 0 0 0 1 2 2 2
  spline S121 degree 2 poles (4.26, -26.4554) (4.4183, -26.1849) (4.6294, -26.0414) (4.768, -26.0414) knots 0 0 0 1 2 2 2
  spline S122 degree 2 poles (4.768, -26.0414) (4.9576, -26.0414) (5.2199, -26.3334) (5.2199, -26.5791) knots 0 0 0 1 2 2 2
  spline S123 degree 2 poles (5.2199, -26.5791) (5.2199, -26.7375) (5.1671, -26.8958) knots 0 0 0 1 1 1
  line L310 (5.1671, -26.8958) -> (5.0368, -26.8958)
  spline S124 degree 2 poles (5.0368, -26.8958) (5.1077, -26.7391) (5.1077, -26.5626) knots 0 0 0 1 1 1
  spline S125 degree 2 poles (5.1077, -26.5626) (5.1077, -26.3812) (4.9247, -26.1684) (4.7828, -26.1684) knots 0 0 0 1 2 2 2
  spline S126 degree 2 poles (4.7828, -26.1684) (4.6476, -26.1684) (4.4859, -26.3136) (4.3474, -26.5544) knots 0 0 0 1 2 2 2
  spline S127 degree 2 poles (4.3474, -26.5544) (4.2055, -26.8034) (3.9862, -26.9684) (3.8427, -26.9684) knots 0 0 0 1 2 2 2
  spline S128 degree 2 poles (3.8427, -26.9684) (3.6382, -26.9684) (3.3809, -26.6847) (3.3809, -26.4257) knots 0 0 0 1 2 2 2
  spline S129 degree 2 poles (3.3809, -26.4257) (3.3809, -26.3334) (3.4369, -26.0942) (3.4749, -26.0316) knots 0 0 0 1 2 2 2
  line L311 (3.4122, -28.5089) -> (3.9664, -28.3044)
  line L312 (3.9664, -28.3044) -> (3.9664, -27.5325)
  line L313 (3.9664, -27.5325) -> (3.4122, -27.3279)
  line L314 (3.4122, -27.3279) -> (3.4122, -27.1927)
  line L315 (3.4122, -27.1927) -> (5.1902, -27.864)
  line L316 (5.1902, -27.864) -> (5.1902, -27.9811)
  line L317 (5.1902, -27.9811) -> (3.4122, -28.6458)
  line L318 (3.4122, -28.6458) -> (3.4122, -28.5089)
  spline S130 degree 2 poles (4.8999, -27.9613) (4.9379, -27.9481) (4.9741, -27.9399) knots 0 0 0 1 1 1
  spline S131 degree 2 poles (4.9741, -27.9399) (5.0038, -27.93) (5.0352, -27.9201) knots 0 0 0 1 1 1
  line L319 (5.0352, -27.9201) -> (5.0352, -27.9151)
  spline S132 degree 2 poles (5.0352, -27.9151) (4.9527, -27.8937) (4.9032, -27.8739) knots 0 0 0 1 1 1
  line L320 (4.9032, -27.8739) -> (4.0785, -27.5753)
  line L321 (4.0785, -27.5753) -> (4.0785, -28.2615)
  line L322 (4.0785, -28.2615) -> (4.8999, -27.9613)
  point P0 (0, 0)
  constraints: 3 equal length, 2 end point, 1 horizontal, 2 other
emboss "Emboss1" sketch "Sketch3" operation cut depth 0.5 direction (-1, 0, 0) wrap yes faces at (-13.3252, 6.2, -2.1656)
thread "Thread1" size "1/4-20 UNC" class "3B" standard "ANSI Unified Screw Threads" length 8.001 offset 3.5
body "Solid1"
